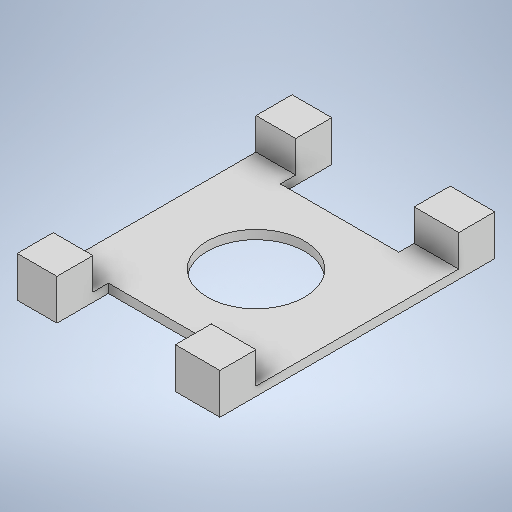
# Autodesk Inventor part: Cover
Saved by Autodesk Inventor 2027 (Build 310192060, 192F)
## iProperties
Created: 2026-07-06
Part Number: Cover
Material: Generic
Document SubType Name: Modeling
Designer: 13129
Density: 1 g/cm^3
Appearance: Default
Author: 13129
Autodesk Inventor part; units mm, degrees
ref_plane "YZ Plane" through (0, 0, 0) normal (1, 0, 0) x (0, 1, 0)
ref_plane "XZ Plane" through (0, 0, 0) normal (0, 1, 0) x (-1, 0, 0)
ref_plane "XY Plane" through (0, 0, 0) normal (0, 0, 1) x (1, 0, 0)
sketch "Sketch1" plane through (0, 0, 0) normal (0, 1, 0) x (-1, 0, 0)
  circle A0 centre (0, 0) radius 12
  line L0 (25, -21.2) -> (-25, -21.2)
  line L1 (25, -21.2) -> (25, 21.2)
  line L2 (25, 21.2) -> (-25, 21.2)
  line L3 (-25, 21.2) -> (-25, -21.2)
  line L4 (25, 21.2) -> (25, 25)
  line L5 (15.2, 21.2) -> (15.2, 25)
  line L6 (25, -21.2) -> (25, -25)
  line L7 (15.2, -21.2) -> (15.2, -25)
  line L8 (25, -25) -> (15.2, -25)
  line L9 (25, 25) -> (15.2, 25)
  line L10 (-25, 21.2) -> (-25, 25)
  line L11 (-14, 21.2) -> (-14, 25)
  line L12 (-25, -21.2) -> (-25, -25)
  line L13 (-14, -21.2) -> (-14, -25)
  line L14 (-14, -25) -> (-25, -25)
  line L15 (-14, 25) -> (-25, 25)
  point P0 (25, 0)
  point P1 (0, -21.2)
  dimension "d0" = 24
  dimension "d4" = 50
  dimension "d5" = 42.4
  dimension "d8" = 9.8
  dimension "d10" = 50
  dimension "d11" = 11
  constraints: 32 end point, 7 vertical, 5 equal length, 5 horizontal, 4 horizontal alignment, 4 perpendicular, 4 point on line, 2 midpoint, 2 vertical alignment, 1 centre point, 1 coincident
  measures "d0" diameter of A0
  measures "d4" distance of L0.start L0.end
  measures "d5" distance of L0.start L1.end
  measures "d8" distance between parallel lines of L4 L5
  measures "d10" distance of L6.end L4.end
  measures "d11" distance of L11.end L10.end
extrude "Extrusion1" add sketch "Sketch1" along normal blind 2.2
sketch "Sketch2" plane through (0, 0, 0) normal (0, -1, 0) x (1, 0, 0)
  line L0 (25, 25) -> (25, -25) construction
  line L1 (-25, 25) -> (-15.2, 25) construction
  line L2 (-15.2, -25) -> (-25, -25) construction
  line L3 (25, -25) -> (14, -25) construction
  line L4 (-25, 25) -> (-15.2, 25)
  line L5 (-25, -25) -> (-15.2, -25)
  line L6 (25, -25) -> (14, -25) construction
  line L7 (14, -25) -> (25, -25)
  line L8 (14, 25) -> (25, 25) construction
  line L9 (14, 25) -> (25, 25)
  line L10 (-25, 25) -> (-25, 33.89)
  line L11 (-25, 33.89) -> (-15.2, 33.89)
  line L12 (-15.2, 33.89) -> (-15.2, 25)
  line L13 (14, 25) -> (14, 33.89)
  line L14 (14, 33.89) -> (25, 33.89)
  line L15 (25, 33.89) -> (25, 25)
  line L16 (-15.2, -25) -> (-25, -25) construction
  line L17 (-25, -25) -> (-25, -33.89)
  line L18 (-25, -33.89) -> (-15.2, -33.89)
  line L19 (-15.2, -33.89) -> (-15.2, -25)
  line L20 (14, -25) -> (14, -33.89)
  line L21 (14, -33.89) -> (25, -33.89)
  line L22 (25, -33.89) -> (25, -25)
  dimension "d12" = 8.89
  dimension "d13" = 8.89
  dimension "d14" = 8.89
  dimension "d15" = 8.89
  constraints: 32 end point, 7 perpendicular, 4 vertical, 3 equal length, 2 horizontal, 1 point on line
  measures "d12" distance of L1.start L10.end
  measures "d13" distance of L8.start L13.end
  measures "d14" distance of L2.end L17.end
  measures "d15" distance between parallel lines of L21 L3
extrude "Extrusion2" add sketch "Sketch2" against normal blind 10
body "Solid1"
